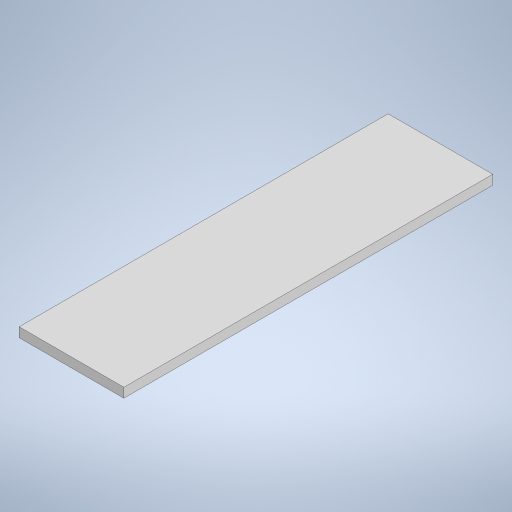
# Autodesk Inventor part: uchwyt_li_pol
Saved by Autodesk Inventor 2023 (Build 270158000, 158)
## iProperties
Created: 2024-08-04
Part Number: uchwyt_li_pol
Material: Ogólny
Document SubType Name: Modeling
Designer: kamil
Density: 1 g/cm^3
Appearance: Domyślna
Author: kamil
Autodesk Inventor part; units mm, degrees
ref_plane "YZ Plane" through (0, 0, 0) normal (1, 0, 0) x (0, 1, 0)
ref_plane "XZ Plane" through (0, 0, 0) normal (0, 1, 0) x (-1, 0, 0)
ref_plane "XY Plane" through (0, 0, 0) normal (0, 0, 1) x (1, 0, 0)
sketch "Szkic7" plane through (0, 0, 0) normal (0, 1, 0) x (-1, 0, 0)
  line L0 (11.5107, 17.5498) -> (-32.4893, 17.5498)
  line L1 (-32.4893, 17.5498) -> (-32.4893, -137.4502)
  line L2 (-32.4893, -137.4502) -> (11.5107, -137.4502)
  line L3 (11.5107, -137.4502) -> (11.5107, 17.5498)
  point P0 (0, 0)
  dimension "d19" = 44
  dimension "d20" = 155
  constraints: 8 end point, 2 parallel, 1 horizontal, 1 perpendicular
  measures "d19" distance of L2.end L1.end
  measures "d20" distance of L1.end L0.end
extrude "Wyciągnięcie proste7" add sketch "Szkic7" along normal blind 4
